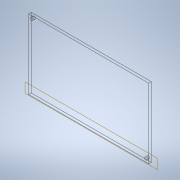
# Autodesk Inventor part: CoverPSU
Saved by Autodesk Inventor 2022.2 (Build 262287000, 287)
## iProperties
Created: 2022-01-15
Part Number: CoverPSU
Material: Generic
Document SubType Name: Modeling
Designer: siwat
Density: 1 g/cm^3
Appearance: Default
Author: siwat
Autodesk Inventor part; units mm, degrees
ref_plane "YZ Plane" through (0, 0, 0) normal (1, 0, 0) x (0, 1, 0)
ref_plane "XZ Plane" through (0, 0, 0) normal (0, 1, 0) x (-1, 0, 0)
ref_plane "XY Plane" through (0, 0, 0) normal (0, 0, 1) x (1, 0, 0)
ref_plane "Work Plane1" through (0, 0, 0) normal (0, 0, 1) x (1, 0, 0)
sketch "Sketch1" plane through (0, 0, 0) normal (0, 0, 1) x (1, 0, 0)
  line L0 (68.1073, 1.6851) -> (-68.1493, 1.6851)
  line L1 (-68.1493, 1.6851) -> (-68.1493, 80.8436)
  line L2 (-68.1493, 80.8436) -> (68.1073, 80.8436)
  line L3 (68.1073, 80.8436) -> (68.1073, 1.6851)
  circle A0 centre (64.7007, 5.0684) radius 1.5
  circle A1 centre (-64.8473, 77.3169) radius 1.5
  point P0 (0, 0)
  dimension "d0" = 3
  dimension "d1" = 3
  constraints: 8 end point, 2 centre point, 2 parallel, 1 horizontal, 1 perpendicular
  measures "d0" diameter of A0
  measures "d1" diameter of A1
extrude "Extrusion1" add sketch "Sketch1" along normal blind 3
body "Solid1"
